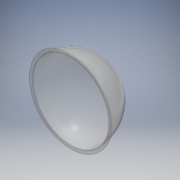
# Autodesk Inventor part: Dome
Saved by Autodesk Inventor 2016 (Build 200138000, 138)
## iProperties
Created: 2016-01-13
Part Number: Dome
Material: Polycarbonate, Clear
Document SubType Name: Modeling
Designer: Conor Mow-Lowry
Density: 1.2 g/cm^3
Appearance: Polycarbonate - Clear
Author: Conor Mow-Lowry
Autodesk Inventor part; units mm, degrees
ref_plane "YZ Plane" through (0, 0, 0) normal (1, 0, 0) x (0, 1, 0)
ref_plane "XZ Plane" through (0, 0, 0) normal (0, 1, 0) x (-1, 0, 0)
ref_plane "XY Plane" through (0, 0, 0) normal (0, 0, 1) x (1, 0, 0)
sketch "Sketch1" plane through (0, 0, 0) normal (0, 1, 0) x (-1, 0, 0)
  arc A0 (295, 0) -> (-295, 0) centre (0, 0) ccw
  arc A1 (299, 0) -> (-299, 0) centre (0, 0) ccw
  line L0 (299, 0) -> (-299, 0)
  dimension "d0" = 590
  dimension "d1" = 598
  constraints: 4 point on circle, 2 centre point, 2 coincident, 2 end point, 2 point on line, 1 horizontal
  measures "d0" diameter of A0
  measures "d1" diameter of A1
revolve "Revolution1" add sketch "Sketch1" angle 180 about axis through (-299, 0, 0) along (-1, 0, 0) contours A0 L0 A1
sketch "Sketch2" plane through (0, 0, 0) normal (0, -1, 0) x (1, 0, 0)
  circle A0 centre (0, 0) radius 295 projected
  circle A1 centre (0, 0) radius 299 projected
  circle A2 centre (0, 0) radius 295
  circle A3 centre (0, 0) radius 322.5
  dimension "d3" = 645
  constraints: 2 centre point, 2 coincident, 1 concentric
  measures "d3" diameter of A3
extrude "Extrusion1" add sketch "Sketch2" along normal blind 4 contours A1 | A3
fillet "Fillet1" radius 2 1 edges at (-295, -4, 0)
fillet "Fillet2" radius 2 2 edges at (0, 0, 299) (0, 0, -299)
body "Solid1"
